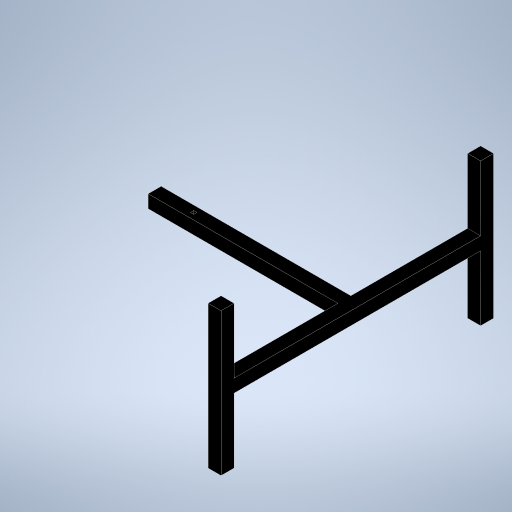
# Autodesk Inventor part: statyw
Saved by Autodesk Inventor 2024 (Build 280153000, 153)
## iProperties
Created: 2024-08-23
Part Number: statyw
Material: Generic
Document SubType Name: Modeling
Designer: domko
Density: 1 g/cm^3
Appearance: Anodized - Black
Author: domko
Autodesk Inventor part; units mm, degrees
ref_plane "YZ Plane" through (0, 0, 0) normal (1, 0, 0) x (0, 1, 0)
ref_plane "XZ Plane" through (0, 0, 0) normal (0, 1, 0) x (-1, 0, 0)
ref_plane "XY Plane" through (0, 0, 0) normal (0, 0, 1) x (1, 0, 0)
sketch "Sketch2" plane through (0, 0, 0) normal (0, 1, 0) x (-1, 0, 0)
  line L0 (150, 10.1481) -> (-142.3178, 10.1481)
  line L1 (-142.3178, -9.8519) -> (150, -9.8519)
  line L2 (150, -9.8519) -> (150, 10.1481)
  line L3 (-142.3178, 10.1481) -> (-142.3178, 210.1481)
  line L4 (-142.3178, 210.1481) -> (-162.3178, 210.1481)
  line L5 (-162.3178, 210.1481) -> (-162.3178, -209.8519)
  line L6 (-162.3178, -209.8519) -> (-142.3178, -209.8519)
  line L7 (-142.3178, -209.8519) -> (-142.3178, -9.8519)
  point P0 (0, 0)
  dimension "d0" = 20
  dimension "d2" = 150
  dimension "d3" = 200
  dimension "d4" = 420
  dimension "d5" = 20
  dimension "d6" = 292.3178
  dimension "d7" = 20
  constraints: 16 end point, 3 perpendicular, 2 vertical, 1 horizontal, 1 parallel, 1 point on line
  measures "d0" distance of L1.end L0.start
  measures "d2" distance from line of point (0, 0) L2
  measures "d3" distance of L6.end L1.start
  measures "d4" distance of L4.end L5.end
  measures "d5" distance of L3.end L4.end
  measures "d6" distance of L1.start L1.end
  measures "d7" distance between parallel lines of L1 L0
extrude "Extrusion1" add sketch "Sketch2" along normal blind 20
sketch "Sketch3" plane through (142.3178, 0, -209.8519) normal (-1, 0, 0) x (0, 0, 1)
  line L0 (0, 120) -> (20, 120)
  line L1 (20, 120) -> (20, -100)
  line L2 (20, -100) -> (0, -100)
  line L3 (0, -100) -> (0, 120)
  line L4 (0, 0) -> (200, 0) projected
  line L5 (0, 20) -> (200, 20) projected
  line L6 (420, -100) -> (400, -100)
  line L7 (400, -100) -> (400, 120)
  line L8 (400, 120) -> (420, 120)
  line L9 (420, 120) -> (420, -100)
  line L10 (420, 0) -> (420, 20) projected
  line L11 (220, 0) -> (420, 0) projected
  line L12 (220, 20) -> (420, 20) projected
  point P0 (209.8519, 0)
  point P1 (400, 20)
  point P2 (400, 0)
  dimension "d10" = 100
  dimension "d11" = 100
  dimension "d12" = 20
  dimension "d13" = 20
  dimension "d14" = 0
  dimension "d15" = 100
  dimension "d16" = 100
  constraints: 16 end point, 4 parallel, 2 horizontal, 2 perpendicular
  measures "d10" distance between parallel lines of L2 L4
  measures "d11" distance between parallel lines of L0 L5
  measures "d12" distance between parallel lines of L3 L1
  measures "d13" distance of L7.end L8.end
  measures "d14" distance between parallel lines of L10 L9
  measures "d15" distance between parallel lines of L11 L6
  measures "d16" distance between parallel lines of L12 L8
extrude "Extrusion2" add sketch "Sketch3" against normal blind 20 contours L0 L1 L5 L3 | L5 L1 L4 L3 | L4 L1 L2 L3 | L6 L7 L11 L9 | L12 L7 L8 L9
sketch "Sketch8" plane through (0, 20, 0) normal (0, 1, 0) x (1, 0, 0)
  line L0 (-150, 9.8519) -> (-150, -10.1481) projected
  line L1 (-92.5, -2.5) -> (-87.5, -2.5)
  line L2 (-87.5, -2.5) -> (-87.5, 2.5)
  line L3 (-87.5, 2.5) -> (-92.5, 2.5)
  line L4 (-92.5, 2.5) -> (-92.5, -2.5)
  point P0 (0, 0)
  point P1 (-90, 0)
  point P2 (-150, -0.1481)
  point P3 (-90, -2.5)
  point P4 (-87.5, 0)
  dimension "d36" = 60
  dimension "d37" = 2.5
  dimension "d38" = 5
  dimension "d39" = 5
  dimension "d40" = 2.5
  constraints: 8 end point, 3 midpoint, 2 parallel, 1 horizontal, 1 perpendicular
  measures "d36" horizontal distance of point (-90, 0) point (-150, -0.148)
  measures "d37" distance of point (-90, -2.5) point (-90, 0)
  measures "d38" distance of L3.end L1.start
  measures "d39" distance of L1.start L1.end
  measures "d40" distance of point (-87.5, 0) point (-90, 0)
extrude "Extrusion4" cut sketch "Sketch8" against normal through all
body "Solid1"
